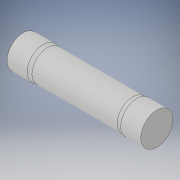
# Autodesk Inventor part: Axel Mk2
Saved by Autodesk Inventor 2019 (Build 230136000, 136)
## iProperties
Created: 2019-02-10
Part Number: Axel Mk2
Material: Generic
Document SubType Name: Modeling
Designer: Kepler
Density: 1 g/cm^3
Appearance: Default
Author: Kepler
Autodesk Inventor part; units mm, degrees
ref_plane "YZ Plane" through (0, 0, 0) normal (1, 0, 0) x (0, 1, 0)
ref_plane "XZ Plane" through (0, 0, 0) normal (0, 1, 0) x (-1, 0, 0)
ref_plane "XY Plane" through (0, 0, 0) normal (0, 0, 1) x (1, 0, 0)
sketch "Sketch1" plane through (0, 0, 0) normal (0, 0, 1) x (1, 0, 0)
  line L0 (0, 0) -> (20, 0)
  line L1 (0, 0) -> (0, -2.4)
  line L2 (0, -2.4) -> (3, -2.4)
  line L3 (3, -2.4) -> (3, -2.3)
  line L4 (3, -2.3) -> (17, -2.3)
  line L5 (17, -2.3) -> (17, -2.4)
  line L6 (17, -2.4) -> (20, -2.4)
  line L7 (20, -2.4) -> (20, 0)
  dimension "d0" = 20
  dimension "d1" = 2.4
  dimension "d7" = 3
  dimension "d8" = 0.1
  dimension "d9" = 14
  dimension "d10" = 0.1
  dimension "d11" = 3
  constraints: 16 end point, 3 perpendicular, 2 horizontal, 1 parallel, 1 vertical
  measures "d0" distance of L0.start L0.end
  measures "d1" distance of L0.start L1.end
  measures "d7" distance of L1.end L2.end
  measures "d8" distance of L2.end L3.end
  measures "d9" distance of L3.end L4.end
  measures "d10" distance of L4.end L5.end
  measures "d11" distance of L5.end L6.end
revolve "Revolution1" add sketch "Sketch1" angle 360 about axis through (0, 0, 0) along (1, 0, 0)
fillet "Fillet1" radius 2 1 edges at (17, 2.3, 0)
fillet "Fillet2" radius 2 1 edges at (3, 2.3, 0)
body "Solid1"
